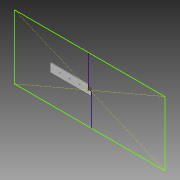
# Autodesk Inventor part: SensorLid
Saved by Autodesk Inventor 2020 (Build 240168000, 168)
## iProperties
Created: 2020-12-18
Part Number: SensorLid
Material: Generic
Document SubType Name: Modeling
Designer: DDeGo
Density: 1 g/cm^3
Appearance: Default
Author: DDeGo
Autodesk Inventor part; units mm, degrees
ref_plane "YZ Plane" through (0, 0, 0) normal (1, 0, 0) x (0, 1, 0)
ref_plane "XZ Plane" through (0, 0, 0) normal (0, 1, 0) x (-1, 0, 0)
ref_plane "XY Plane" through (0, 0, 0) normal (0, 0, 1) x (1, 0, 0)
sketch "Sketch1" plane through (0, 0, 0) normal (0, 0, 1) x (1, 0, 0)
  line L0 (122, -13.5) -> (-122, -13.5)
  line L1 (-122, -13.5) -> (-122, 13.5)
  line L2 (-122, 13.5) -> (122, 13.5)
  line L3 (122, 13.5) -> (122, -13.5)
  line L4 (122, -13.5) -> (-122, 13.5) construction
  line L5 (-122, -13.5) -> (122, 13.5) construction
  line L6 (0, 0) -> (-31, 0) construction
  circle A0 centre (-93, 0) radius 1.4
  circle A1 centre (-62, 0) radius 1.4
  circle A2 centre (-31, 0) radius 1.4
  circle A3 centre (0, 0) radius 1.4
  circle A4 centre (31, 0) radius 1.4
  circle A5 centre (62, 0) radius 1.4
  circle A6 centre (93, 0) radius 1.4
  dimension "d0" = 27
  dimension "d1" = 244
  dimension "d2" = 2.8
  dimension "d5" = 31
  dimension "d10" = 31
  constraints: 14 end point, 7 centre point, 3 horizontal, 2 coincident, 2 midpoint, 2 parallel, 1 perpendicular, 12 other
  measures "d0" distance of L0.end L1.end
  measures "d1" distance of L1.end L2.end
  measures "d2" diameter of A0
  measures "d5" distance of A0.centre A1.centre
  measures "d10" distance of L6.start L6.end
extrude "Extrusion1" add sketch "Sketch1" along normal blind 2 contours L0 L1 L2 L3 | A3
sketch "Sketch2" plane through (0, 0, 2) normal (0, 0, 1) x (1, 0, 0)
  line L0 (-5, 99.1699) -> (-5, 0)
  line L1 (-5, 0) -> (5, 0)
  line L2 (5, 0) -> (5, -99.1699)
  line L3 (232.2267, -99.1699) -> (-232.2267, -99.1699)
  line L4 (-232.2267, -99.1699) -> (-232.2267, 99.1699)
  line L5 (-232.2267, 99.1699) -> (232.2267, 99.1699)
  line L6 (232.2267, 99.1699) -> (232.2267, -99.1699)
  line L7 (232.2267, -99.1699) -> (-232.2267, 99.1699) construction
  line L8 (-232.2267, -99.1699) -> (232.2267, 99.1699) construction
  point P0 (0, 0)
  dimension "d13" = 10
  constraints: 18 end point, 4 perpendicular, 3 midpoint, 2 parallel, 2 point on line, 1 horizontal, 1 vertical
  measures "d13" distance of L0.end L1.end
extrude "Extrusion2" cut sketch "Sketch2" against normal through all contours L5 L6 L3 L2 L1 L0
body "Solid1"
